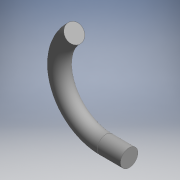
# Autodesk Inventor part: ValveRing0
Saved by Autodesk Inventor 2018 (Build 220112000, 112)
## iProperties
Created: 2018-10-01
Part Number: ValveRing0
Material: Generic
Document SubType Name: Modeling
Designer: Isaac Newcomb
Density: 1 g/cm^3
Appearance: Default
Author: Isaac Newcomb
Autodesk Inventor part; units mm, degrees
ref_plane "YZ Plane" through (0, 0, 0) normal (1, 0, 0) x (0, 1, 0)
ref_plane "XZ Plane" through (0, 0, 0) normal (0, 1, 0) x (-1, 0, 0)
ref_plane "XY Plane" through (0, 0, 0) normal (0, 0, 1) x (1, 0, 0)
sketch "Sweep Path" plane through (0, 0, 0) normal (1, 0, 0) x (0, 1, 0)
  arc A0 (5.8535, 5.4531) -> (-8, 0) centre (0, 0) ccw
  line L0 (0, 0) -> (5.8535, 5.4531) construction
  line L1 (0, 0) -> (8, 0) construction
  line L2 (0, 0) -> (-8, 0) construction
  dimension "d0" = 8
  dimension "d1" = 42.972
  constraints: 6 end point, 2 horizontal, 2 point on circle, 1 centre point, 1 coincident, 1 equal length
  measures "d0" radius of A0
  measures "d1" angle of L1 L0
sketch "Sweep Profile" plane through (0, 0, 0) normal (0, 0, 1) x (1, 0, 0)
  circle A0 centre (0, -8) radius 1.5
  point P0 (0, 0)
  dimension "d2" = 3
  constraints: 1 centre point, 1 coincident
  measures "d2" diameter of A0
sweep "Ring" add profiles "Sweep Profile" path "Sweep Path"
sketch "Sketch4" plane through (0, -8, 0) normal (0, 0, -1) x (-1, 0, 0)
  circle A0 centre (0, 0) radius 1.5 projected
  point P0 (0, 8)
extrude "Extrusion2" add sketch "Sketch4" along normal blind 4
equation "\"d0\" = SweepRadius"
equation "\"d1\" = SweepAngle"
equation "\"d2\" = RingThickness"
equation "\"RingDiameter\" = 4"
equation "\"SweepRadius\" = 8"
equation "\"SweepAngle\" = 42.971835deg"
equation "\"RingThickness\" = 3"
body "Solid1"
